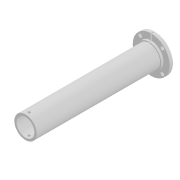
# Autodesk Inventor part: Coil_Stand
Saved by Autodesk Inventor 2022.1 (Build 261234000, 234)
## iProperties
Created: 2022-06-17
Part Number: Coil_Stand
Material: Generic
Document SubType Name: Modeling
Designer: william
Density: 1 g/cm^3
Appearance: Default
Author: william
Autodesk Inventor part; units mm, degrees
ref_plane "YZ Plane" through (0, 0, 0) normal (1, 0, 0) x (0, 1, 0)
ref_plane "XZ Plane" through (0, 0, 0) normal (0, 1, 0) x (-1, 0, 0)
ref_plane "XY Plane" through (0, 0, 0) normal (0, 0, 1) x (1, 0, 0)
sketch "Sketch1" plane through (0, 0, 0) normal (0, 0, 1) x (1, 0, 0)
  circle A0 centre (0, 0) radius 10
  circle A1 centre (0, 0) radius 8
  dimension "d0" = 20
  dimension "d1" = 2
  constraints: 2 centre point, 2 coincident
  measures "d0" diameter of A0
  measures "d1" radial gap between concentric circles of A0 A1
extrude "Extrusion1" add sketch "Sketch1" along normal blind 115
sketch "Sketch2" plane through (0, 0, 0) normal (0, 0, -1) x (-1, 0, 0)
  circle A0 centre (0, 0) radius 16.5
  circle A1 centre (0, 0) radius 8
  circle A2 centre (0, 0) radius 8 construction
  dimension "d4" = 33
  constraints: 3 coincident, 2 centre point, 1 concentric
  measures "d4" diameter of A0
extrude "Extrusion2" add sketch "Sketch2" against normal blind 3
sketch "Sketch3" plane through (0, 0, 3) normal (0, 0, 1) x (1, 0, 0)
  circle A0 centre (9.8995, 9.8995) radius 1.55
  line L0 (9.8995, 9.8995) -> (0, 0) construction
  line L1 (0, 0) -> (4.9931, 0) construction
  dimension "d7" = 14
  dimension "d8" = 3.1
  dimension "d14" = 45
  constraints: 4 end point, 1 centre point, 1 horizontal
  measures "d7" distance of L0.end L0.start
  measures "d8" diameter of A0
  measures "d14" angle of L1 L0
extrude "Extrusion3" cut sketch "Sketch3" against normal through all
sketch "Sketch7" plane through (0, 0, 3) normal (0, 0, 1) x (1, 0, 0)
  circle A0 centre (0, 0) radius 11
  circle A1 centre (0, 0) radius 10
  circle A2 centre (0, 0) radius 10 construction
  dimension "d30" = 1
  constraints: 2 centre point, 2 coincident, 1 concentric
  measures "d30" radial gap between concentric circles of A0 A1
extrude "Extrusion7" add sketch "Sketch7" along normal blind 2
pattern_circular "Circular Pattern1" count 4 over 360 about axis through (0, 0, 0) along (0, 0, 1) of "Extrusion3"
sketch "Sketch5" plane through (0, 0, 3) normal (0, 0, 1) x (1, 0, 0)
  line L0 (-0.5, 10) -> (0.5, 10)
  line L1 (0.5, 10) -> (0.5, 20)
  line L2 (0.5, 20) -> (-0.5, 20)
  line L3 (-0.5, 20) -> (-0.5, 10)
  line L4 (-0.5, 10) -> (0.5, 20) construction
  line L5 (0.5, 10) -> (-0.5, 20) construction
  point P0 (0, 0)
  point P1 (0, 15)
  point P2 (0, 15)
  dimension "d21" = 1
  dimension "d22" = 10
  dimension "d23" = 10
  constraints: 12 end point, 3 midpoint, 2 parallel, 1 horizontal, 1 perpendicular, 1 vertical alignment
  measures "d21" distance of L1.end L2.end
  measures "d22" distance from line of point (0, 0) L0
  measures "d23" distance of L2.end L0.start
extrude "Extrusion5" cut sketch "Sketch5" along normal blind 2 and the other way blind 2
sketch "Sketch6" plane through (0, 0, 0) normal (0, 1, 0) x (-1, 0, 0)
  circle A0 centre (0, 112) radius 1.25
  line L0 (10, 115) -> (-10, 115) construction
  point P0 (0, 0)
  dimension "d26" = 3
  dimension "d27" = 2.5
  constraints: 1 centre point, 1 vertical alignment
  measures "d26" distance from line of L0 A0.centre
  measures "d27" diameter of A0
extrude "Extrusion6" cut sketch "Sketch6" along normal through all both and the other way through all
body "Solid1"
